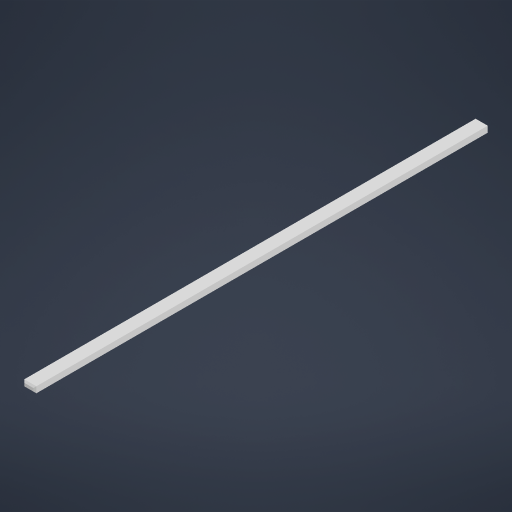
# Autodesk Inventor part: Elbow_Both_Rod_V1
Saved by Autodesk Inventor 2024.1 (Build 281209000, 209)
## iProperties
Created: 2023-07-01
Part Number: Elbow_Both_Rod_V1
Material: Generic
Document SubType Name: Modeling
Designer: User
Density: 1 g/cm^3
Appearance: Default
Author: User
Autodesk Inventor part; units mm, degrees
ref_plane "YZ Plane" through (0, 0, 0) normal (1, 0, 0) x (0, 1, 0)
ref_plane "XZ Plane" through (0, 0, 0) normal (0, 1, 0) x (-1, 0, 0)
ref_plane "XY Plane" through (0, 0, 0) normal (0, 0, 1) x (1, 0, 0)
sketch "Sketch1" plane through (0, 0, 0) normal (0, 0, 1) x (1, 0, 0)
  line L0 (0, 0) -> (-8, 0)
  line L1 (-8, 0) -> (-8, 4)
  line L2 (-8, 4) -> (0, 4)
  line L3 (0, 4) -> (0, 0)
  dimension "d0" = 8
  dimension "d1" = 4
  constraints: 8 end point, 2 parallel, 1 horizontal, 1 perpendicular
  measures "d0" distance of L1.end L2.end
  measures "d1" distance of L0.end L1.end
extrude "Extrusion1" add sketch "Sketch1" along normal blind 300
chamfer "Chamfer1" distance 1 angle 45 4 edges at (-4, 4, 300) (0, 2, 300) (-4, 0, 300) (-8, 2, 300)
chamfer "Chamfer2" distance 1 angle 45 4 edges at (-4, 4, 0) (0, 2, 0) (-4, 0, 0) (-8, 2, 0)
body "Solid1"
